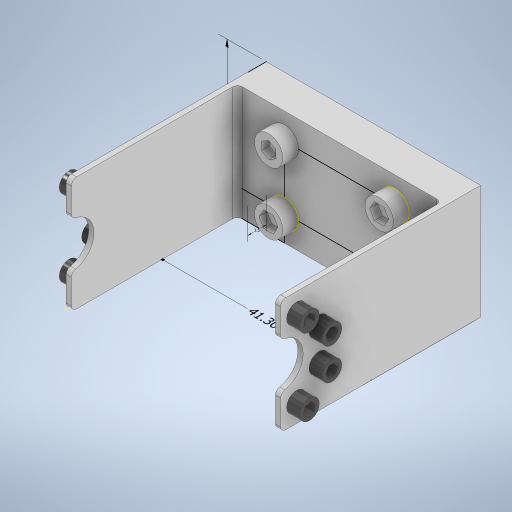
# Autodesk Inventor part: link_manip_parafusos
Saved by Autodesk Inventor 2024 (Build 280153000, 153)
## iProperties
Created: 2024-10-15
Part Number: link_manip_parafusos
Material: Genérico
Document SubType Name: Modeling
Designer: robof
Density: 1 g/cm^3
Appearance: Padrão
Author: robof
Autodesk Inventor part; units mm, degrees
ref_plane "YZ Plane" through (0, 0, 0) normal (1, 0, 0) x (0, 1, 0)
ref_plane "XZ Plane" through (0, 0, 0) normal (0, 1, 0) x (-1, 0, 0)
ref_plane "XY Plane" through (0, 0, 0) normal (0, 0, 1) x (1, 0, 0)
sketch "Esboço1" plane through (0, 0, 0) normal (0, 1, 0) x (-1, 0, 0)
  line L0 (0, 0) -> (-41.3, 0)
  line L1 (-41.3, 0) -> (-41.3, -35)
  line L2 (-41.3, -35) -> (0, -35)
  line L3 (0, -35) -> (0, 0)
  dimension "d0" = 41.3
  dimension "d1" = 35
  constraints: 8 end point, 2 parallel, 1 horizontal, 1 perpendicular
  measures "d0" distance of L2.end L1.end
  measures "d1" distance of L1.end L0.end
extrude "Extrusão1" add sketch "Esboço1" along normal blind 35
sketch "Esboço2" plane through (0, 35, 0) normal (0, 1, 0) x (1, 0, 0)
  line L0 (0, 35) -> (0, 0) projected
  line L1 (0, 35) -> (1, 35)
  line L2 (1, 35) -> (1, 32)
  line L3 (1, 32) -> (0, 32)
  line L4 (0, 32) -> (0, 35)
  line L5 (41.3, 0) -> (41.3, 35) projected
  line L6 (41.3, 0) -> (40.3, 0)
  line L7 (40.3, 0) -> (40.3, 3)
  line L8 (40.3, 3) -> (41.3, 3)
  line L9 (41.3, 3) -> (41.3, 0)
  line L10 (40.3, 3) -> (1, 3)
  line L11 (1, 3) -> (1, 32)
  line L12 (1, 32) -> (40.3, 32)
  line L13 (40.3, 32) -> (40.3, 3)
  line L14 (40.3, 3) -> (1, 3)
  line L15 (1, 3) -> (1, 0)
  line L16 (1, 0) -> (40.3, 0)
  line L17 (40.3, 0) -> (40.3, 3)
  point P0 (1, 3)
  dimension "d4" = 1
  dimension "d5" = 3
  dimension "d6" = 1
  dimension "d7" = 3
  constraints: 32 end point, 8 parallel, 4 horizontal, 4 perpendicular, 2 point on line
  measures "d4" distance of L2.end L3.end
  measures "d5" distance of L1.end L2.end
  measures "d6" distance of L7.end L8.end
  measures "d7" distance of L6.end L7.end
extrude "Extrusão2" cut sketch "Esboço2" against normal blind 35 contours L12 L13 L10 L11 | L10 L7 L16 L15
sketch "Esboço3" plane through (41.3, 0, 0) normal (1, 0, 0) x (0, 0, -1)
  line L0 (0, 0) -> (0, 35) projected
  line L1 (32, 0) -> (0, 0) projected
  line L2 (35, 0) -> (35, 35) projected
  line L3 (0, 0) -> (35, 0)
  line L4 (35, 0) -> (35, 22)
  line L5 (35, 22) -> (0, 22)
  line L6 (0, 22) -> (0, 0)
  line L7 (0, 22) -> (35, 22)
  line L8 (35, 22) -> (35, 35)
  line L9 (35, 35) -> (0, 35)
  line L10 (0, 35) -> (0, 22)
  dimension "d11" = 22
  constraints: 16 end point, 4 parallel, 2 horizontal, 2 perpendicular, 2 point on line
  measures "d11" distance of L4.end L3.end
extrude "Extrusão3" cut sketch "Esboço3" against normal blind 65 contours L0 L9 L2 L5
sketch "Esboço4" plane through (41.3, 0, 0) normal (1, 0, 0) x (0, 0, -1)
  line L0 (0, 0) -> (0, 22) projected
  circle A0 centre (0, 11) radius 4
  circle A1 centre (0, 11) radius 7.99
  line L1 (0, 11) -> (3.0576, 18.3818)
  line L2 (0, 11) -> (7.99, 11) construction
  circle A2 centre (3.0576, 18.3818) radius 1.9
  circle A3 centre (-3.0576, 18.3818) radius 1.9
  circle A4 centre (-7.3818, 14.0576) radius 1.9
  circle A5 centre (-7.3818, 7.9424) radius 1.9
  circle A6 centre (-3.0576, 3.6182) radius 1.9
  circle A7 centre (3.0576, 3.6182) radius 1.9
  circle A8 centre (7.3818, 7.9424) radius 1.9
  circle A9 centre (7.3818, 14.0576) radius 1.9
  dimension "d15" = 15.98
  dimension "d14" = 8
  dimension "d16" = 67.5
  dimension "d17" = 3.8
  dimension "d20" = 360
  constraints: 9 centre point, 4 end point, 2 coincident, 1 equal length, 1 horizontal, 1 midpoint, 20 other
  measures "d14" diameter of A0
  measures "d16" angle of L2 L1
  measures "d17" diameter of A2
extrude "Extrusão4" add sketch "Esboço4" along normal blind 2.5 contours A7 A1 | A1 A7 | A8 A1 | A1 A8 | A2 A1 L1 | L1 A1 A2 | A2 A1 | A9 A1 | A1 A9
sketch "Esboço5" plane through (43.8, 18.3818, -3.0576) normal (1, 0, 0) x (0, 0, -1)
  line L0 (-0.0101, -1.2843) -> (-1.1173, -0.6334)
  line L1 (-1.1173, -0.6334) -> (-1.1072, 0.6509)
  line L2 (-1.1072, 0.6509) -> (0.0101, 1.2843)
  line L3 (0.0101, 1.2843) -> (1.1173, 0.6334)
  line L4 (1.1173, 0.6334) -> (1.1072, -0.6509)
  line L5 (1.1072, -0.6509) -> (-0.0101, -1.2843)
  line L6 (-3.0576, -18.3818) -> (-3.0576, 3.6182) projected
  circle A0 centre (-3.0576, -7.3818) radius 4.35
  point P0 (0, 0)
  point P1 (-3.0576, -3.0318)
  point P2 (-3.0576, -11.7318)
  dimension "d24" = 8.7
  constraints: 12 end point, 1 centre point, 1 midpoint, 13 other
  measures "d24" diameter of A0
extrude "Extrusão5" add sketch "Esboço5" against normal blind 20 contours L6 A0 picked at (-2.4285, -6.0754)
sketch "Esboço6" plane through (43.8, 18.3818, -3.0576) normal (1, 0, 0) x (0, 0, -1)
  arc A0 (-3.0576, -11.7318) -> (-3.0576, -3.0318) centre (-3.0576, -7.3818) ccw projected
  circle A1 centre (-3.0576, -7.3818) radius 4.35
  point P0 (-3.0576, -18.3818)
  point P1 (-3.0576, -3.0318)
  constraints: 1 centre point, 1 coincident
extrude "Extrusão6" cut sketch "Esboço6" against normal blind 100
sketch "Esboço7" plane through (43.8, 18.3818, -3.0576) normal (1, 0, 0) x (0, 0, -1)
  line L0 (-0.0047, -1.2049) -> (-1.0458, -0.5984)
  line L1 (-1.0458, -0.5984) -> (-1.0411, 0.6065)
  line L2 (-1.0411, 0.6065) -> (0.0047, 1.2049)
  line L3 (0.0047, 1.2049) -> (1.0458, 0.5984)
  line L4 (1.0458, 0.5984) -> (1.0411, -0.6065)
  line L5 (1.0411, -0.6065) -> (-0.0047, -1.2049)
  arc A0 (-3.0576, -11.7318) -> (-3.0576, -3.0318) centre (-3.0576, -7.3818) ccw projected
  circle A1 centre (-3.0576, -7.3818) radius 4.35
  line L6 (-5.2666, -0.8553) -> (-6.4317, -1.1626)
  line L7 (-6.4317, -1.1626) -> (-7.2803, -0.3073)
  line L8 (-7.2803, -0.3073) -> (-6.9639, 0.8553)
  line L9 (-6.9639, 0.8553) -> (-5.7989, 1.1626)
  line L10 (-5.7989, 1.1626) -> (-4.9502, 0.3073)
  line L11 (-4.9502, 0.3073) -> (-5.2666, -0.8553)
  line L12 (-9.2346, -4.3289) -> (-9.8411, -5.37)
  line L13 (-9.8411, -5.37) -> (-11.046, -5.3653)
  line L14 (-11.046, -5.3653) -> (-11.6443, -4.3194)
  line L15 (-11.6443, -4.3194) -> (-11.0378, -3.2783)
  line L16 (-11.0378, -3.2783) -> (-9.8329, -3.2831)
  line L17 (-9.8329, -3.2831) -> (-9.2346, -4.3289)
  line L18 (-9.5841, -9.5908) -> (-9.2768, -10.7558)
  line L19 (-9.2768, -10.7558) -> (-10.1321, -11.6045)
  line L20 (-10.1321, -11.6045) -> (-11.2948, -11.2881)
  line L21 (-11.2948, -11.2881) -> (-11.602, -10.123)
  line L22 (-11.602, -10.123) -> (-10.7467, -9.2744)
  line L23 (-10.7467, -9.2744) -> (-9.5841, -9.5908)
  line L24 (-6.1106, -13.5587) -> (-5.0695, -14.1652)
  line L25 (-5.0695, -14.1652) -> (-5.0742, -15.3701)
  line L26 (-5.0742, -15.3701) -> (-6.12, -15.9685)
  line L27 (-6.12, -15.9685) -> (-7.1611, -15.362)
  line L28 (-7.1611, -15.362) -> (-7.1564, -14.1571)
  line L29 (-7.1564, -14.1571) -> (-6.1106, -13.5587)
  line L30 (-0.8486, -13.9083) -> (0.3164, -13.601)
  line L31 (0.3164, -13.601) -> (1.165, -14.4563)
  line L32 (1.165, -14.4563) -> (0.8486, -15.6189)
  line L33 (0.8486, -15.6189) -> (-0.3164, -15.9262)
  line L34 (-0.3164, -15.9262) -> (-1.165, -15.0709)
  line L35 (-1.165, -15.0709) -> (-0.8486, -13.9083)
  line L36 (3.1193, -10.4347) -> (3.7258, -9.3936)
  line L37 (3.7258, -9.3936) -> (4.9307, -9.3983)
  line L38 (4.9307, -9.3983) -> (5.529, -10.4442)
  line L39 (5.529, -10.4442) -> (4.9225, -11.4853)
  line L40 (4.9225, -11.4853) -> (3.7176, -11.4805)
  line L41 (3.7176, -11.4805) -> (3.1193, -10.4347)
  line L42 (3.4688, -5.1728) -> (3.1616, -4.0078)
  line L43 (3.1616, -4.0078) -> (4.0169, -3.1591)
  line L44 (4.0169, -3.1591) -> (5.1795, -3.4755)
  line L45 (5.1795, -3.4755) -> (5.4868, -4.6406)
  line L46 (5.4868, -4.6406) -> (4.6314, -5.4892)
  line L47 (4.6314, -5.4892) -> (3.4688, -5.1728)
  point P0 (-3.0576, -18.3818)
  point P1 (0, 0)
  point P2 (-6.1153, 0)
  point P3 (-10.4394, -4.3242)
  point P4 (-10.4394, -10.4394)
  point P5 (-6.1153, -14.7636)
  point P6 (0, -14.7636)
  point P7 (4.3242, -10.4394)
  point P8 (4.3242, -4.3242)
  dimension "d31" = 360
  constraints: 96 end point, 1 centre point, 1 coincident, 118 other
extrude "Extrusão7" cut sketch "Esboço7" against normal blind 1.5 contours L0 L1 L2 L3 L4 L5 | L30 L31 L32 L33 L34 L35 | L36 L37 L38 L39 L40 L41 | L42 L43 L44 L45 L46 L47
sketch "Esboço8" plane through (0, 0, -35) normal (-1, 0, 0) x (0, 0, 1)
  circle A0 centre (31.9424, 3.6182) radius 1.9 projected
  circle A1 centre (31.9424, 3.6182) radius 1.9
  arc A2 (35, 15.35) -> (35, 6.65) centre (35, 11) ccw projected
  circle A3 centre (35, 11) radius 4.35
  circle A4 centre (38.0576, 3.6182) radius 1.9
  circle A5 centre (42.3818, 7.9424) radius 1.9
  circle A6 centre (42.3818, 14.0576) radius 1.9
  circle A7 centre (38.0576, 18.3818) radius 1.9
  circle A8 centre (31.9424, 18.3818) radius 1.9
  circle A9 centre (27.6182, 14.0576) radius 1.9
  circle A10 centre (27.6182, 7.9424) radius 1.9
  point P0 (35, 0)
  dimension "d37" = 360
  constraints: 9 centre point, 2 coincident, 17 other
extrude "Extrusão8" add sketch "Esboço8" along normal blind 2.5 contours A0 | A8 | A9 | A10
sketch "Esboço9" plane through (-2.5, 7.9424, -7.3818) normal (-1, 0, 0) x (0, 0, 1)
  arc A0 (7.3818, 7.4076) -> (7.3818, -1.2924) centre (7.3818, 3.0576) ccw projected
  circle A1 centre (7.3818, 3.0576) radius 4.35
  circle A2 centre (4.3242, -4.3242) radius 1.9 projected
  line L0 (5.1728, -3.4688) -> (4.0078, -3.1616) projected
  line L1 (4.0078, -3.1616) -> (5.1728, -3.4688)
  line L2 (5.1728, -3.4688) -> (5.4892, -4.6314)
  line L3 (5.4892, -4.6314) -> (4.6406, -5.4868)
  line L4 (4.6406, -5.4868) -> (3.4755, -5.1795)
  line L5 (3.4755, -5.1795) -> (3.1591, -4.0169)
  line L6 (3.1591, -4.0169) -> (4.0078, -3.1616)
  line L7 (9.3936, -3.7258) -> (10.4347, -3.1193)
  line L8 (10.4347, -3.1193) -> (11.4805, -3.7176)
  line L9 (11.4805, -3.7176) -> (11.4853, -4.9225)
  line L10 (11.4853, -4.9225) -> (10.4442, -5.529)
  line L11 (10.4442, -5.529) -> (9.3983, -4.9307)
  line L12 (9.3983, -4.9307) -> (9.3936, -3.7258)
  line L13 (13.601, -0.3164) -> (13.9083, 0.8486)
  line L14 (13.9083, 0.8486) -> (15.0709, 1.165)
  line L15 (15.0709, 1.165) -> (15.9262, 0.3164)
  line L16 (15.9262, 0.3164) -> (15.6189, -0.8486)
  line L17 (15.6189, -0.8486) -> (14.4563, -1.165)
  line L18 (14.4563, -1.165) -> (13.601, -0.3164)
  line L19 (14.1652, 5.0695) -> (13.5587, 6.1106)
  line L20 (13.5587, 6.1106) -> (14.1571, 7.1564)
  line L21 (14.1571, 7.1564) -> (15.362, 7.1611)
  line L22 (15.362, 7.1611) -> (15.9685, 6.12)
  line L23 (15.9685, 6.12) -> (15.3701, 5.0742)
  line L24 (15.3701, 5.0742) -> (14.1652, 5.0695)
  line L25 (10.7558, 9.2768) -> (9.5908, 9.5841)
  line L26 (9.5908, 9.5841) -> (9.2744, 10.7467)
  line L27 (9.2744, 10.7467) -> (10.123, 11.602)
  line L28 (10.123, 11.602) -> (11.2881, 11.2948)
  line L29 (11.2881, 11.2948) -> (11.6045, 10.1321)
  line L30 (11.6045, 10.1321) -> (10.7558, 9.2768)
  line L31 (5.37, 9.8411) -> (4.3289, 9.2346)
  line L32 (4.3289, 9.2346) -> (3.2831, 9.8329)
  line L33 (3.2831, 9.8329) -> (3.2783, 11.0378)
  line L34 (3.2783, 11.0378) -> (4.3194, 11.6443)
  line L35 (4.3194, 11.6443) -> (5.3653, 11.046)
  line L36 (5.3653, 11.046) -> (5.37, 9.8411)
  line L37 (1.1626, 6.4317) -> (0.8553, 5.2666)
  line L38 (0.8553, 5.2666) -> (-0.3073, 4.9502)
  line L39 (-0.3073, 4.9502) -> (-1.1626, 5.7989)
  line L40 (-1.1626, 5.7989) -> (-0.8553, 6.9639)
  line L41 (-0.8553, 6.9639) -> (0.3073, 7.2803)
  line L42 (0.3073, 7.2803) -> (1.1626, 6.4317)
  line L43 (0.5984, 1.0458) -> (1.2049, 0.0047)
  line L44 (1.2049, 0.0047) -> (0.6065, -1.0411)
  line L45 (0.6065, -1.0411) -> (-0.5984, -1.0458)
  line L46 (-0.5984, -1.0458) -> (-1.2049, -0.0047)
  line L47 (-1.2049, -0.0047) -> (-0.6065, 1.0411)
  line L48 (-0.6065, 1.0411) -> (0.5984, 1.0458)
  point P0 (7.3818, -7.9424)
  point P1 (10.4394, -4.3242)
  point P2 (14.7636, 0)
  point P3 (14.7636, 6.1153)
  point P4 (10.4394, 10.4394)
  point P5 (4.3242, 10.4394)
  point P6 (0, 6.1153)
  point P7 (0, 0)
  dimension "d43" = 360
  constraints: 96 end point, 2 coincident, 1 centre point, 118 other
extrude "Extrusão9" cut sketch "Esboço9" against normal blind 1.5 contours L2 L3 L4 L5 L6 L0 | L31 L32 L33 L34 L35 L36 | L37 L38 L39 L40 L41 L42 | L43 L44 L45 L46 L47 L48
fillet "Arredondamento1" radius 1 6 edges at (40.3, 11, -32) (1, 11, -32) (40.8, 15.35, 0) (40.8, 6.65, 0) (0.5, 6.65, 0) (0.5, 15.35, 0)
fillet "Arredondamento2" radius 1 4 edges at (40.8, 0, 0) (0.5, 0, 0) (0.5, 22, 0) (40.8, 22, 0)
sketch "Esboço11" plane through (41.3, 0, -35) normal (0, 0, -1) x (-1, 0, 0)
  line L0 (41.3, 22) -> (0, 22) projected
  line L1 (41.3, 22) -> (31.3, 22)
  line L2 (31.3, 22) -> (36.3, 22)
  line L3 (31.3, 22) -> (26.3, 22)
  line L4 (2, 22) -> (39.3, 22) projected
  line L5 (31.3, 22) -> (31.3, 17)
  circle A0 centre (31.3, 17) radius 2.75
  line L6 (20.65, 22) -> (20.65, 14.25)
  circle A1 centre (10, 17) radius 2.75
  line L7 (0, 6.7267) -> (0, 15.2733) projected
  line L8 (0, 11) -> (12.75, 11)
  circle A2 centre (31.3, 5) radius 2.75
  circle A3 centre (10, 5) radius 2.75
  point P0 (41.3, 0)
  dimension "d58" = 10
  dimension "d59" = 5
  dimension "d60" = 5
  dimension "d61" = 5
  dimension "d62" = 5.5
  constraints: 12 end point, 4 centre point, 3 midpoint, 3 symmetric about line, 2 point on line, 2 vertical, 1 coincident, 1 horizontal, 3 other
  measures "d58" distance of L0.start L1.end
  measures "d59" distance of L1.end L2.end
  measures "d60" distance of L1.end L3.end
  measures "d61" distance of L1.end L5.end
  measures "d62" diameter of A0
extrude "Extrusão10" add sketch "Esboço11" along normal blind 3
sketch "Esboço12" plane through (31.3, 17, -38) normal (0, 0, -1) x (-1, 0, 0)
  line L0 (1.8235, 0.0077) -> (0.9184, -1.5753)
  line L1 (0.9184, -1.5753) -> (-0.9051, -1.5831)
  line L2 (-0.9051, -1.5831) -> (-1.8235, -0.0077)
  line L3 (-1.8235, -0.0077) -> (-0.9184, 1.5753)
  line L4 (-0.9184, 1.5753) -> (0.9051, 1.5831)
  line L5 (0.9051, 1.5831) -> (1.8235, 0.0077)
  line L6 (-10, -17) -> (-10, 5) projected
  line L7 (-10, -6) -> (-2.9592, -6)
  line L8 (-8, -17) -> (29.3, -17) projected
  line L9 (10.65, -17) -> (10.65, -10.3267)
  line L10 (1.8235, -12.0077) -> (0.9184, -10.4247)
  line L11 (0.9184, -10.4247) -> (-0.9051, -10.4169)
  line L12 (-0.9051, -10.4169) -> (-1.8235, -11.9923)
  line L13 (-1.8235, -11.9923) -> (-0.9184, -13.5753)
  line L14 (-0.9184, -13.5753) -> (0.9051, -13.5831)
  line L15 (0.9051, -13.5831) -> (1.8235, -12.0077)
  line L16 (19.4765, 0.0077) -> (20.3816, -1.5753)
  line L17 (20.3816, -1.5753) -> (22.2051, -1.5831)
  line L18 (22.2051, -1.5831) -> (23.1235, -0.0077)
  line L19 (23.1235, -0.0077) -> (22.2184, 1.5753)
  line L20 (22.2184, 1.5753) -> (20.3949, 1.5831)
  line L21 (20.3949, 1.5831) -> (19.4765, 0.0077)
  line L22 (19.4765, -12.0077) -> (20.3816, -10.4247)
  line L23 (20.3816, -10.4247) -> (22.2051, -10.4169)
  line L24 (22.2051, -10.4169) -> (23.1235, -11.9923)
  line L25 (23.1235, -11.9923) -> (22.2184, -13.5753)
  line L26 (22.2184, -13.5753) -> (20.3949, -13.5831)
  line L27 (20.3949, -13.5831) -> (19.4765, -12.0077)
  point P0 (31.3, -17)
  point P1 (0, 0)
  point P2 (0, -12)
  point P3 (21.3, 0)
  point P4 (24.2592, -6)
  point P5 (21.3, -12)
  constraints: 52 end point, 22 symmetric about line, 2 midpoint, 1 horizontal, 1 vertical, 13 other
extrude "Extrusão11" cut sketch "Esboço12" against normal blind 1.5
sketch "Esboço13" plane through (2, 0, -32) normal (0, 0, 1) x (1, 0, 0)
  circle A0 centre (8, 17) radius 2.75 projected
  circle A1 centre (8, 17) radius 2.75
  circle A2 centre (8, 5) radius 2.75 projected
  circle A3 centre (8, 5) radius 2.75
  circle A4 centre (29.3, 5) radius 2.75 projected
  circle A5 centre (29.3, 5) radius 2.75
  circle A6 centre (29.3, 17) radius 2.75
  point P0 (-2, 0)
  constraints: 4 centre point, 3 coincident
extrude "Extrusão12" add sketch "Esboço13" along normal blind 3
sketch "Esboço14" plane through (10, 17, -29) normal (0, 0, 1) x (1, 0, 0)
  line L0 (0.9051, 1.5831) -> (-0.9184, 1.5753) projected
  line L1 (-0.0067, 1.5792) -> (1.3643, 0.7954)
  line L2 (1.3643, 0.7954) -> (1.371, -0.7838)
  line L3 (1.371, -0.7838) -> (0.0067, -1.5792)
  line L4 (0.0067, -1.5792) -> (-1.3643, -0.7954)
  line L5 (-1.3643, -0.7954) -> (-1.371, 0.7838)
  line L6 (-1.371, 0.7838) -> (-0.0067, 1.5792)
  line L7 (-0.9184, -13.5753) -> (0.9051, -13.5831) projected
  line L8 (-0.9184, -13.5753) -> (-1.8236, -12.0078)
  line L9 (-1.8236, -12.0078) -> (-0.9186, -10.4402)
  line L10 (-0.9186, -10.4402) -> (0.8914, -10.4401)
  line L11 (0.8914, -10.4401) -> (1.7966, -12.0076)
  line L12 (1.7966, -12.0076) -> (0.8916, -13.5752)
  line L13 (0.8916, -13.5752) -> (-0.9184, -13.5753)
  circle A0 centre (21.3, -12) radius 2.75 projected
  line L14 (19.4765, -12.0077) -> (20.3949, -13.5831) projected
  line L15 (20.3949, -13.5831) -> (19.4765, -12.0077)
  line L16 (19.4765, -12.0077) -> (20.3816, -10.4247)
  line L17 (20.3816, -10.4247) -> (22.2051, -10.4169)
  line L18 (22.2051, -10.4169) -> (23.1235, -11.9923)
  line L19 (23.1235, -11.9923) -> (22.2184, -13.5753)
  line L20 (22.2184, -13.5753) -> (20.3949, -13.5831)
  circle A1 centre (21.3, 0) radius 2.75 projected
  line L21 (20.3816, -1.5753) -> (22.2051, -1.5831) projected
  line L22 (20.3816, -1.5753) -> (19.4765, 0.0077)
  line L23 (19.4765, 0.0077) -> (20.3949, 1.5831)
  line L24 (20.3949, 1.5831) -> (22.2184, 1.5753)
  line L25 (22.2184, 1.5753) -> (23.1235, -0.0077)
  line L26 (23.1235, -0.0077) -> (22.2051, -1.5831)
  line L27 (22.2051, -1.5831) -> (20.3816, -1.5753)
  point P0 (-10, -17)
  point P1 (0, 0)
  point P2 (-0.0135, -12.0077)
  constraints: 48 end point, 2 coincident, 1 midpoint, 52 other
extrude "Extrusão13" cut sketch "Esboço14" against normal blind 1.5 contours L1 L2 L3 L4 L5 L6 | L8 L9 L10 L11 L12 L13 | L16 L17 L18 L19 L20 L14 | L22 L23 L24 L25 L26 L21
sketch "Esboço15" plane through (0, 0, -35) normal (-1, 0, 0) x (0, 0, 1)
  line L0 (0, 0) -> (0, 22) projected
  line L1 (0, 22) -> (-3.5, 22)
  line L2 (-3.5, 22) -> (-3.5, 0)
  line L3 (-3.5, 0) -> (0, 0)
  line L4 (0, 0) -> (0, 22)
  point P0 (35, 0)
  dimension "d71" = 3.5
  constraints: 8 end point, 2 parallel, 1 horizontal, 1 perpendicular
  measures "d71" distance of L3.end L2.end
sketch "Esboço16" plane through (0, 0, 0) normal (0, -1, 0) x (1, 0, 0)
  line L0 (41.3, -35) -> (0, -35) projected
  line L1 (41.3, -35) -> (0, -35)
  line L2 (0, -35) -> (0, -38.5)
  line L3 (0, -38.5) -> (41.3, -38.5)
  line L4 (41.3, -38.5) -> (41.3, -35)
  point P0 (0, 0)
  dimension "d72" = 3.5
  constraints: 8 end point, 2 parallel, 1 horizontal, 1 perpendicular
  measures "d72" distance of L2.end L1.end
extrude "Extrusão14" add sketch "Esboço16" against normal blind 22
sketch "Esboço17" plane through (2, 0, -32) normal (0, 0, 1) x (1, 0, 0)
  circle A0 centre (8, 5) radius 2.75 projected
  line L0 (-2, 0) -> (8, 0)
  line L1 (8, 0) -> (8, 5)
  line L2 (8, 5) -> (-2, 5)
  line L3 (-2, 5) -> (-2, 0)
  circle A1 centre (29.3, 17) radius 2.75 projected
  line L4 (8, 5) -> (29.3, 5)
  line L5 (29.3, 5) -> (29.3, 17)
  line L6 (29.3, 17) -> (8, 17)
  line L7 (8, 17) -> (8, 5)
  constraints: 16 end point, 4 parallel, 2 horizontal, 2 perpendicular
